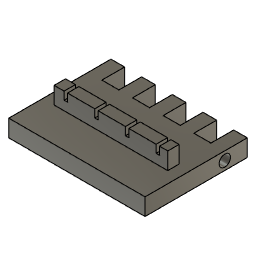
Protohand palm v3 (Autodesk Fusion 360 design; units mm, degrees)
Autodesk Fusion 360 part; units mm, degrees
note: some values were not read from the file. Set by a fixed rule: which sketch regions a step uses.
sketch "Sketch1" plane through (0, 0, 0) normal (0, 0, 1) x (1, 0, 0)
  line L0 (130, 0) -> (130, 50)
  line L1 (130, 50) -> (130, 70)
  line L2 (130, 70) -> (118, 70)
  line L3 (118, 70) -> (118, 50)
  line L4 (118, 50) -> (103, 50)
  line L5 (103, 50) -> (103, 70)
  line L6 (103, 70) -> (91, 70)
  line L7 (91, 70) -> (91, 50)
  line L8 (91, 50) -> (76, 50)
  line L9 (76, 50) -> (76, 70)
  line L10 (76, 70) -> (64, 70)
  line L11 (64, 70) -> (64, 50)
  line L12 (64, 50) -> (49, 50)
  line L13 (49, 50) -> (49, 70)
  line L14 (49, 70) -> (37, 70)
  line L15 (37, 70) -> (37, 50)
  line L16 (37, 50) -> (22, 50)
  line L17 (22, 50) -> (22, 70)
  line L18 (22, 70) -> (10, 70)
  line L19 (10, 70) -> (10, 50)
  line L20 (10, 50) -> (10, 0)
  line L21 (10, 0) -> (10, -20)
  line L22 (10, -20) -> (130, -20)
  line L23 (130, -20) -> (130, 0)
  dimension "d1" = 12
  dimension "d2" = 15
  dimension "d3" = 12
  dimension "d4" = 15
  dimension "d5" = 12
  dimension "d6" = 15
  dimension "d7" = 12
  dimension "d8" = 15
  dimension "d9" = 12
  dimension "d11" = 20
  dimension "d14" = 20
  dimension "d15" = 20
  dimension "d16" = 20
  dimension "d17" = 20
  dimension "d18" = 20
  dimension "d19" = 20
  dimension "d20" = 20
  dimension "d21" = 20
  dimension "d49" = 120
  dimension "d50" = 70
  dimension "d51" = 70
  constraint parallel L0 L1
  constraint perpendicular L0 L2
  constraint perpendicular L2 L3
  constraint perpendicular L3 L4
  constraint perpendicular L4 L5
  constraint perpendicular L3 L6
  constraint perpendicular L6 L7
  constraint perpendicular L3 L8
  constraint perpendicular L8 L9
  constraint perpendicular L9 L10
  constraint perpendicular L10 L11
  constraint perpendicular L11 L12
  constraint perpendicular L12 L13
  constraint perpendicular L13 L14
  constraint perpendicular L12 L15
  constraint perpendicular L15 L16
  constraint perpendicular L16 L17
  constraint perpendicular L15 L18
  constraint perpendicular L18 L19
  constraint parallel L20 L21
  constraint perpendicular L20 L22
  constraint perpendicular L22 L23
  measures "d1" distance of L1.end L2.end
  measures "d2" distance of L3.end L4.end
  measures "d3" distance of L5.end L6.end
  measures "d4" distance of L7.end L8.end
  measures "d5" distance of L9.end L10.end
  measures "d6" distance of L11.end L12.end
  measures "d7" distance of L13.end L14.end
  measures "d8" distance of L15.end L16.end
  measures "d9" distance of L17.end L18.end
  measures "d11" distance of L0.end L1.end
  measures "d14" distance of L18.end L19.end
  measures "d15" distance of L16.end L17.end
  measures "d16" distance of L14.end L15.end
  measures "d17" distance of L12.end L13.end
  measures "d18" distance of L10.end L11.end
  measures "d19" distance of L8.end L9.end
  measures "d20" distance of L6.end L7.end
  measures "d21" distance of L4.end L5.end
  measures "d49" distance of L21.end L22.end
  measures "d50" distance of L0.end L22
  measures "d51" distance of L19.end L22
extrude "Extrude1" add sketch "Sketch1" along normal blind 15
hole "Hole1" at (10, 50.1961, 7.5484) direction (1, 0, 0) diameter 10 depth 120 tip angle 180
sketch "Sketch2" plane through (0, 0, 15) normal (0, 0, 1) x (-1, 0, 0)
  line L0 (-130, 20) -> (-130, -70)
  line L1 (-130, -70) -> (-118, -70)
  line L2 (-118, -70) -> (-118, -50)
  line L3 (-118, -50) -> (-103, -50)
  line L4 (-103, -50) -> (-103, -70)
  line L5 (-103, -70) -> (-91, -70)
  line L6 (-91, -70) -> (-91, -50)
  line L7 (-91, -50) -> (-76, -50)
  line L8 (-76, -50) -> (-76, -70)
  line L9 (-76, -70) -> (-64, -70)
  line L10 (-64, -70) -> (-64, -50)
  line L11 (-64, -50) -> (-49, -50)
  line L12 (-49, -50) -> (-49, -70)
  line L13 (-49, -70) -> (-37, -70)
  line L14 (-37, -70) -> (-37, -50)
  line L15 (-37, -50) -> (-22, -50)
  line L16 (-22, -50) -> (-22, -70)
  line L17 (-22, -70) -> (-10, -70)
  line L18 (-10, -70) -> (-10, 20)
  line L19 (-20, -20) -> (-120, -20)
  line L20 (-120, -20) -> (-120, -10)
  line L21 (-120, -10) -> (-20, -10)
  line L22 (-20, -10) -> (-20, -20)
  line L23 (-10, 20) -> (-130, 20)
  dimension "d28" = 100
  dimension "d29" = 10
  constraint horizontal L19
  constraint vertical L20
  constraint horizontal L21
  constraint vertical L22
  measures "d28" distance of L20.end L21.end
  measures "d29" distance of L19.end L20.end
extrude "Extrude2" add sketch "Sketch2" along normal blind 15 contours L19 L20 L21 L22
sketch "Sketch3" plane through (0, 20, 0) normal (0, 1, 0) x (-1, 0, 0)
  line L0 (-120, 15) -> (-20, 15)
  line L1 (-20, 15) -> (-20, 30)
  line L2 (-20, 30) -> (-120, 30)
  line L3 (-120, 30) -> (-120, 15)
  line L4 (-112.7366, 30) -> (-109.7366, 30)
  line L5 (-109.7366, 30) -> (-109.7366, 23)
  line L6 (-109.7366, 23) -> (-112.7366, 23)
  line L7 (-112.7366, 23) -> (-112.7366, 30)
  line L8 (-85.7366, 30) -> (-82.7366, 30)
  line L9 (-82.7366, 30) -> (-82.7366, 23)
  line L10 (-82.7366, 23) -> (-85.7366, 23)
  line L11 (-85.7366, 23) -> (-85.7366, 30)
  line L12 (-58.7366, 30) -> (-55.7366, 30)
  line L13 (-55.7366, 30) -> (-55.7366, 23)
  line L14 (-55.7366, 23) -> (-58.7366, 23)
  line L15 (-58.7366, 23) -> (-58.7366, 30)
  line L16 (-31.7366, 30) -> (-28.7366, 30)
  line L17 (-28.7366, 30) -> (-28.7366, 23)
  line L18 (-28.7366, 23) -> (-31.7366, 23)
  line L19 (-31.7366, 23) -> (-31.7366, 30)
  dimension "d32" = 7
  dimension "d33" = 3
  dimension "d34" = 7
  dimension "d35" = 3
  dimension "d36" = 7
  dimension "d37" = 3
  dimension "d38" = 7
  dimension "d39" = 3
  dimension "d40" = 24
  dimension "d41" = 24
  dimension "d42" = 24
  dimension "d43" = 7.2634
  constraint horizontal L4
  constraint vertical L5
  constraint horizontal L6
  constraint vertical L7
  constraint coincident L2 L4.start
  constraint horizontal L8
  constraint vertical L9
  constraint horizontal L10
  constraint vertical L11
  constraint coincident L2 L8.start
  constraint horizontal L12
  constraint vertical L13
  constraint horizontal L14
  constraint vertical L15
  constraint coincident L2 L12.start
  constraint horizontal L16
  constraint vertical L17
  constraint horizontal L18
  constraint vertical L19
  constraint coincident L2 L16.start
  measures "d32" distance of L4.start L6.end
  measures "d33" distance of L5 L7
  measures "d34" distance of L8.start L10.end
  measures "d35" distance of L9 L11
  measures "d36" distance of L12.start L14.end
  measures "d37" distance of L13 L15
  measures "d38" distance of L16.start L18.end
  measures "d39" distance of L17 L19
  measures "d40" distance of L5 L11
  measures "d41" distance of L9 L15
  measures "d42" distance of L13 L19
  measures "d43" distance of L3 L7
extrude "Extrude3" cut sketch "Sketch3" against normal blind 20 contours L2 L4 L5 L6 L7 | L2 L16 L17 L18 L19 | L2 L8 L9 L10 L11 | L2 L12 L13 L14 L15
sketch "Sketch4" plane through (0, 0, 15) normal (0, 0, 1) x (-1, 0, 0)
  line L0 (-20, -10) -> (-20, -20)
  line L1 (-20, -20) -> (-120, -20)
  line L2 (-120, -20) -> (-120, -10)
  line L3 (-120, -10) -> (-20, -10)
  line L4 (-130, 20) -> (-130, -70)
  line L5 (-130, -70) -> (-118, -70)
  line L6 (-118, -70) -> (-118, -50)
  line L7 (-118, -50) -> (-103, -50)
  line L8 (-103, -50) -> (-103, -70)
  line L9 (-103, -70) -> (-91, -70)
  line L10 (-91, -70) -> (-91, -50)
  line L11 (-91, -50) -> (-76, -50)
  line L12 (-76, -50) -> (-76, -70)
  line L13 (-76, -70) -> (-64, -70)
  line L14 (-64, -70) -> (-64, -50)
  line L15 (-64, -50) -> (-49, -50)
  line L16 (-49, -50) -> (-49, -70)
  line L17 (-49, -70) -> (-37, -70)
  line L18 (-37, -70) -> (-37, -50)
  line L19 (-37, -50) -> (-22, -50)
  line L20 (-22, -50) -> (-22, -70)
  line L21 (-22, -70) -> (-10, -70)
  line L22 (-10, -70) -> (-10, 20)
  line L23 (-10, 20) -> (-130, 20)
